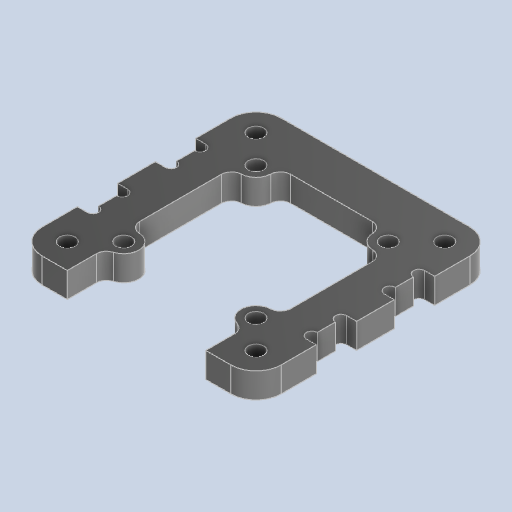
# Autodesk Inventor part: Head_camera_frame
Saved by Autodesk Inventor 2022.5 (Build 265521000, 521)
## iProperties
Created: 2023-04-07
Part Number: Head_camera_frame
Material: アセタール樹脂、黒
Document SubType Name: Modeling
Designer: Masato Kubotera
Density: 1.425 g/cm^3
Appearance: 滑らか - 黒
Description: POM T5
Author: Masato Kubotera
Revision Number: Rev.2 Specifications for RoboCup 2023: Changed design to reduce tilt error by reducing the number of parts at the joint between the camera and the neck.
Autodesk Inventor part; units mm, degrees
ref_plane "YZ Plane" through (0, 0, 0) normal (1, 0, 0) x (0, 1, 0)
ref_plane "XZ Plane" through (0, 0, 0) normal (0, 1, 0) x (-1, 0, 0)
ref_plane "XY Plane" through (0, 0, 0) normal (0, 0, 1) x (1, 0, 0)
derived "e-CAM50_CUNX.ipt"
sketch "スケッチ1" plane through (0, 0, 0) normal (0, 0, 1) x (1, 0, 0)
  line L0 (-15, -15) -> (15, -15)
  line L1 (15, -15) -> (15, 15)
  line L2 (15, 15) -> (-15, 15)
  line L3 (-15, 15) -> (-15, -15)
  line L4 (-15, -15) -> (15, 15) construction
  line L5 (15, -15) -> (-15, 15) construction
  line L6 (-15, 0) -> (15, 0) construction
  line L7 (0, 15) -> (0, -15) construction
  line L8 (-13.14, 13.14) -> (13.14, 13.14) construction
  line L9 (13.14, 13.14) -> (13.14, -13.14) construction
  line L10 (13.14, -13.14) -> (-13.14, -13.14) construction
  line L11 (-13.14, -13.14) -> (-13.14, 13.14) construction
  line L12 (-13.14, 13.14) -> (13.14, -13.14) construction
  line L13 (13.14, 13.14) -> (-13.14, -13.14) construction
  circle A0 centre (0, 0) radius 8.5
  line L14 (-7, 8) -> (7, 8)
  line L15 (8, 7) -> (8, -7)
  line L16 (7, -8) -> (-7, -8)
  line L17 (-8, -7) -> (-8, 7)
  line L18 (-8, 8) -> (8, -8) construction
  line L19 (8, 8) -> (-8, -8) construction
  arc A1 (-8, -7) -> (-7, -8) centre (-7, -7) ccw
  arc A2 (7, -8) -> (8, -7) centre (7, -7) ccw
  arc A3 (8, 7) -> (7, 8) centre (7, 7) ccw
  arc A4 (-7, 8) -> (-8, 7) centre (-7, 7) ccw
  arc A5 (-2, -10) -> (2, -10) centre (0, -10) ccw
  line L20 (-2, -10) -> (-2, -8)
  line L21 (2, -10) -> (2, -8)
  line L22 (-2, 10) -> (-2, 8)
  arc A6 (2, 10) -> (-2, 10) centre (0, 10) ccw
  line L23 (2, 10) -> (2, 8)
  circle A7 centre (-13.14, -13.14) radius 1.1
  circle A8 centre (13.14, -13.14) radius 1.1
  circle A9 centre (-13.14, 13.14) radius 1.1
  circle A10 centre (13.14, 13.14) radius 1.1
  circle A11 centre (-13.14, -13.14) radius 2 construction
  circle A12 centre (13.14, -13.14) radius 2 construction
  circle A13 centre (-13.14, 13.14) radius 2 construction
  circle A14 centre (13.14, 13.14) radius 2 construction
  arc A15 (-10.219, -12.456) -> (-12.456, -10.219) centre (-13.14, -13.14) ccw
  line L24 (-14, -8.2717) -> (-14, 8.2717)
  line L25 (-8.2717, -14) -> (8.2717, -14)
  arc A16 (-14, -8.2717) -> (-12.456, -10.219) centre (-12, -8.2717) ccw
  arc A17 (-10.219, -12.456) -> (-8.2717, -14) centre (-8.2717, -12) ccw
  arc A18 (-12.456, 10.219) -> (-14, 8.2717) centre (-12, 8.2717) ccw
  arc A19 (-12.456, 10.219) -> (-10.219, 12.456) centre (-13.14, 13.14) ccw
  arc A20 (-8.2717, 14) -> (-10.219, 12.456) centre (-8.2717, 12) ccw
  line L26 (-8.2717, 14) -> (8.2717, 14)
  arc A21 (8.2717, -14) -> (10.219, -12.456) centre (8.2717, -12) ccw
  arc A22 (12.456, -10.219) -> (10.219, -12.456) centre (13.14, -13.14) ccw
  arc A23 (12.456, -10.219) -> (14, -8.2717) centre (12, -8.2717) ccw
  line L27 (14, -8.2717) -> (14, 8.2717)
  arc A24 (14, 8.2717) -> (12.456, 10.219) centre (12, 8.2717) ccw
  arc A25 (10.219, 12.456) -> (12.456, 10.219) centre (13.14, 13.14) ccw
  arc A26 (10.219, 12.456) -> (8.2717, 14) centre (8.2717, 12) ccw
  point P0 (-10.2659, -14)
  point P1 (-14, -10.2659)
sketch "スケッチ2" plane through (0, 0, 0) normal (0, 0, 1) x (1, 0, 0)
  line L0 (-15, 0) -> (15, 0) construction
  line L1 (0, 15) -> (0, -15) construction
  circle A0 centre (-13.14, -13.14) radius 1.55
  circle A1 centre (13.14, -13.14) radius 1.55
  circle A2 centre (13.14, 13.14) radius 1.55
  circle A3 centre (-13.14, 13.14) radius 1.55
  line L2 (18.75, -23.75) -> (-18.75, -23.75)
  line L3 (-23.75, -18.75) -> (-23.75, 18.75)
  line L4 (-18.75, 23.75) -> (18.75, 23.75)
  line L5 (23.75, 18.75) -> (23.75, -18.75)
  line L6 (23.75, -23.75) -> (-23.75, 23.75) construction
  line L7 (-23.75, -23.75) -> (23.75, 23.75) construction
  arc A4 (-23.75, -18.75) -> (-18.75, -23.75) centre (-18.75, -18.75) ccw
  arc A5 (18.75, -23.75) -> (23.75, -18.75) centre (18.75, -18.75) ccw
  arc A6 (23.75, 18.75) -> (18.75, 23.75) centre (18.75, 18.75) ccw
  arc A7 (-18.75, 23.75) -> (-23.75, 18.75) centre (-18.75, 18.75) ccw
  line L8 (-11.75, -23.75) -> (-11.75, -21.75)
  line L9 (-9.55, -21.75) -> (-5.95, -21.75)
  arc A8 (-9.55, -21.75) -> (-11.75, -21.75) centre (-10.65, -21.75) ccw
  line L10 (-7.75, -21.75) -> (-7.75, -23.75) construction
  line L11 (-3.75, -23.75) -> (-3.75, -21.75)
  arc A9 (-3.75, -21.75) -> (-5.95, -21.75) centre (-4.85, -21.75) ccw
  line L12 (11.75, -23.75) -> (11.75, -21.75)
  line L13 (9.55, -21.75) -> (5.95, -21.75)
  arc A10 (11.75, -21.75) -> (9.55, -21.75) centre (10.65, -21.75) ccw
  line L14 (3.75, -23.75) -> (3.75, -21.75)
  arc A11 (5.95, -21.75) -> (3.75, -21.75) centre (4.85, -21.75) ccw
  line L15 (-11.75, 23.75) -> (-11.75, 21.75)
  line L16 (-9.55, 21.75) -> (-5.95, 21.75)
  arc A12 (-11.75, 21.75) -> (-9.55, 21.75) centre (-10.65, 21.75) ccw
  line L17 (-3.75, 23.75) -> (-3.75, 21.75)
  arc A13 (-5.95, 21.75) -> (-3.75, 21.75) centre (-4.85, 21.75) ccw
  line L18 (11.75, 23.75) -> (11.75, 21.75)
  arc A14 (9.55, 21.75) -> (11.75, 21.75) centre (10.65, 21.75) ccw
  line L19 (9.55, 21.75) -> (5.95, 21.75)
  line L20 (3.75, 23.75) -> (3.75, 21.75)
  arc A15 (3.75, 21.75) -> (5.95, 21.75) centre (4.85, 21.75) ccw
  circle A16 centre (-18.75, -18.75) radius 1.55
  circle A17 centre (-18.75, -18.75) radius 3 construction
  arc A18 (-18.75, -23.75) -> (-23.75, -18.75) centre (-18.75, -18.75) ccw construction
  circle A19 centre (18.75, -18.75) radius 1.55
  circle A20 centre (18.75, -18.75) radius 3 construction
  circle A21 centre (-18.75, 18.75) radius 1.55
  circle A22 centre (-18.75, 18.75) radius 3 construction
  circle A23 centre (18.75, 18.75) radius 3 construction
  circle A24 centre (18.75, 18.75) radius 1.55
  arc A25 (23.75, -18.75) -> (18.75, -23.75) centre (18.75, -18.75) ccw construction
  line L21 (23.75, -13.75) -> (17.9429, -13.75)
  arc A26 (16.0217, -12.306) -> (10.1412, -13.056) centre (13.14, -13.14) ccw
  line L22 (8.142, -15) -> (-8.142, -15)
  arc A27 (-10.1412, -13.056) -> (-13.056, -10.1412) centre (-13.14, -13.14) ccw
  line L23 (-15, -8.142) -> (-15, 8.142)
  line L24 (23.75, 13.75) -> (17.9429, 13.75)
  arc A28 (10.1412, 13.056) -> (16.0217, 12.306) centre (13.14, 13.14) ccw
  line L25 (8.142, 15) -> (-8.142, 15)
  arc A29 (-13.056, 10.1412) -> (-10.1412, 13.056) centre (-13.14, 13.14) ccw
  line L26 (-15, 15) -> (-15, -15) projected
  line L27 (-15, -15) -> (15, -15) projected
  arc A30 (16.0217, -12.306) -> (17.9429, -13.75) centre (17.9429, -11.75) ccw
  arc A31 (8.142, -15) -> (10.1412, -13.056) centre (8.142, -13) ccw
  arc A32 (-10.1412, -13.056) -> (-8.142, -15) centre (-8.142, -13) ccw
  arc A33 (-15, -8.142) -> (-13.056, -10.1412) centre (-13, -8.142) ccw
  arc A34 (-13.056, 10.1412) -> (-15, 8.142) centre (-13, 8.142) ccw
  arc A35 (-8.142, 15) -> (-10.1412, 13.056) centre (-8.142, 13) ccw
  arc A36 (10.1412, 13.056) -> (8.142, 15) centre (8.142, 13) ccw
  arc A37 (17.9429, 13.75) -> (16.0217, 12.306) centre (17.9429, 11.75) ccw
  point P0 (0, 0)
  point P1 (0, 0)
  point P2 (11.75, -23.75)
  point P3 (11.75, 23.75)
  point P4 (3.75, 23.75)
  point P5 (-3.75, 23.75)
  point P6 (-11.75, 23.75)
  point P7 (16.0773, -13.75)
  point P8 (10.7862, -15)
  point P9 (-10.7862, -15)
  point P10 (-15, -10.7862)
  point P11 (-15, 10.7862)
  point P12 (16.0773, 13.75)
  point P13 (16.0773, 13.75)
  point P14 (10.7862, 15)
  point P15 (-10.7862, 15)
  dimension "d1" = 3.1
  dimension "d2" = 3.1
  dimension "d3" = 3.1
  dimension "d4" = 3.1
  dimension "d5" = 47.5
  dimension "d6" = 47.5
  dimension "d7" = 5
  dimension "d9" = 1.1
  dimension "d10" = 2
  dimension "d12" = 8
  dimension "d13" = 7.5
  dimension "d14" = 3.1
  dimension "d15" = 6
  dimension "d18" = 3
  dimension "d19" = 3
  dimension "d20" = 2
  dimension "d21" = 2
  constraints: 60 point on circle, 48 end point, 42 symmetric about line, 38 centre point, 26 tangent, 23 point on line, 12 coincident, 10 equal radius, 3 horizontal, 3 midpoint, 3 parallel, 2 collinear, 2 perpendicular, 2 vertical, 16 other
  measures "d1" diameter of A0
  measures "d2" diameter of A1
  measures "d3" diameter of A2
  measures "d4" diameter of A3
  measures "d5" distance of L6.end L7.end
  measures "d6" distance of L7.start L6.end
  measures "d7" radius of A4
  measures "d9" radius of A8
  measures "d10" distance of L8.start L8.end
  measures "d12" distance between parallel lines of L11 L8
  measures "d13" distance between parallel lines of L14 L11
  measures "d14" diameter of A16
  measures "d15" diameter of A17
  measures "d18" radius of A27
  measures "d19" radius of A26
  measures "d20" radius of A30
  measures "d21" distance edge to line of A18 L8
extrude "押し出し1" add sketch "スケッチ2" along normal blind 5 contours L2 L12 A10 L13 A11 L14 L11 A9 L9 A8 L8 A4 L3 A7 L4 L15 A12 L16 A13 L17 L20 A15 L19 A14 L18 A6 L5 L24 A37 A28 A36 L25 A35 A29 A34 L23 L26 L27 L22 A31 A26 A30 L21 A5 | L27 L26 A33 A27 A32
equation "\"d6\" = d5"
equation "\"d19\" = d18"
